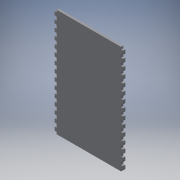
# Autodesk Inventor part: дно
Saved by Autodesk Inventor 2019 (Build 230136000, 136)
## iProperties
Created: 2022-02-24
Part Number: дно
Material: Типовые
Document SubType Name: Modeling
Designer: korsh
Density: 1 g/cm^3
Appearance: По умолчанию
Author: korsh
Autodesk Inventor part; units mm, degrees
ref_plane "YZ Plane" through (0, 0, 0) normal (1, 0, 0) x (0, 1, 0)
ref_plane "XZ Plane" through (0, 0, 0) normal (0, 1, 0) x (-1, 0, 0)
ref_plane "XY Plane" through (0, 0, 0) normal (0, 0, 1) x (1, 0, 0)
sketch "Эскиз1" plane through (0, 0, 0) normal (0, 0, 1) x (1, 0, 0)
  line L0 (0, 180) -> (0, 170) projected
  line L1 (0, 180) -> (-6, 180) projected
  line L2 (-6, 170) -> (-6, 180) projected
  line L3 (0, 170) -> (-6, 170) projected
  line L4 (0, 160) -> (0, 150) projected
  line L5 (0, 160) -> (-6, 160) projected
  line L6 (-6, 150) -> (-6, 160) projected
  line L7 (0, 150) -> (-6, 150) projected
  line L8 (0, 140) -> (0, 130) projected
  line L9 (0, 140) -> (-6, 140) projected
  line L10 (-6, 130) -> (-6, 140) projected
  line L11 (0, 130) -> (-6, 130) projected
  line L12 (0, 120) -> (0, 110) projected
  line L13 (0, 120) -> (-6, 120) projected
  line L14 (-6, 110) -> (-6, 120) projected
  line L15 (0, 110) -> (-6, 110) projected
  line L16 (0, 100) -> (0, 90) projected
  line L17 (0, 100) -> (-6, 100) projected
  line L18 (-6, 90) -> (-6, 100) projected
  line L19 (0, 90) -> (-6, 90) projected
  line L20 (0, 80) -> (0, 70) projected
  line L21 (0, 80) -> (-6, 80) projected
  line L22 (-6, 70) -> (-6, 80) projected
  line L23 (0, 70) -> (-6, 70) projected
  line L24 (0, 60) -> (0, 50) projected
  line L25 (0, 60) -> (-6, 60) projected
  line L26 (-6, 50) -> (-6, 60) projected
  line L27 (0, 50) -> (-6, 50) projected
  line L28 (0, 40) -> (0, 30) projected
  line L29 (0, 40) -> (-6, 40) projected
  line L30 (-6, 30) -> (-6, 40) projected
  line L31 (0, 30) -> (-6, 30) projected
  line L32 (0, 20) -> (0, 10) projected
  line L33 (0, 20) -> (-6, 20) projected
  line L34 (-6, 10) -> (-6, 20) projected
  line L35 (0, 10) -> (-6, 10) projected
  line L36 (0, 0) -> (0, -10) projected
  line L37 (0, 0) -> (-6, 0) projected
  line L38 (-6, -10) -> (-6, 0) projected
  line L39 (0, -10) -> (-6, -10) projected
  line L40 (0, -20) -> (0, -30) projected
  line L41 (0, -20) -> (-6, -20) projected
  line L42 (-6, -30) -> (-6, -20) projected
  line L43 (0, -30) -> (-6, -30) projected
  line L44 (0, -20) -> (0, -30) projected
  line L45 (0, -20) -> (-6, -20) projected
  line L46 (-6, -30) -> (-6, -20) projected
  line L47 (0, -30) -> (-6, -30) projected
  line L48 (0, -40) -> (0, -50) projected
  line L49 (0, -40) -> (-6, -40) projected
  line L50 (-6, -50) -> (-6, -40) projected
  line L51 (0, -50) -> (-6, -50) projected
  line L52 (0, -60) -> (0, -70) projected
  line L53 (0, -60) -> (-6, -60) projected
  line L54 (-6, -70) -> (-6, -60) projected
  line L55 (0, -70) -> (-6, -70) projected
  line L56 (0, -80) -> (0, -90) projected
  line L57 (0, -80) -> (-6, -80) projected
  line L58 (-6, -90) -> (-6, -80) projected
  line L59 (0, -90) -> (-6, -90) projected
  line L60 (0, -100) -> (0, -110) projected
  line L61 (0, -100) -> (-6, -100) projected
  line L62 (-6, -110) -> (-6, -100) projected
  line L63 (0, -110) -> (-6, -110) projected
  line L64 (-186, 180) -> (-186, 170) projected
  line L65 (-186, 180) -> (-192, 180) projected
  line L66 (-192, 170) -> (-192, 180) projected
  line L67 (-186, 170) -> (-192, 170) projected
  line L68 (-186, 160) -> (-186, 150) projected
  line L69 (-186, 160) -> (-192, 160) projected
  line L70 (-192, 150) -> (-192, 160) projected
  line L71 (-186, 150) -> (-192, 150) projected
  line L72 (-186, 140) -> (-186, 130) projected
  line L73 (-186, 140) -> (-192, 140) projected
  line L74 (-192, 130) -> (-192, 140) projected
  line L75 (-186, 130) -> (-192, 130) projected
  line L76 (-186, 120) -> (-186, 110) projected
  line L77 (-186, 120) -> (-192, 120) projected
  line L78 (-192, 110) -> (-192, 120) projected
  line L79 (-186, 110) -> (-192, 110) projected
  line L80 (-186, 100) -> (-186, 90) projected
  line L81 (-186, 100) -> (-192, 100) projected
  line L82 (-192, 90) -> (-192, 100) projected
  line L83 (-186, 90) -> (-192, 90) projected
  line L84 (-186, 80) -> (-186, 70) projected
  line L85 (-186, 80) -> (-192, 80) projected
  line L86 (-192, 70) -> (-192, 80) projected
  line L87 (-186, 70) -> (-192, 70) projected
  line L88 (-186, 60) -> (-186, 50) projected
  line L89 (-186, 60) -> (-192, 60) projected
  line L90 (-192, 50) -> (-192, 60) projected
  line L91 (-186, 50) -> (-192, 50) projected
  line L92 (-186, 20) -> (-186, 10) projected
  line L93 (-186, 20) -> (-192, 20) projected
  line L94 (-192, 10) -> (-192, 20) projected
  line L95 (-186, 10) -> (-192, 10) projected
  line L96 (-186, 40) -> (-186, 30) projected
  line L97 (-186, 40) -> (-192, 40) projected
  line L98 (-192, 30) -> (-192, 40) projected
  line L99 (-186, 30) -> (-192, 30) projected
  line L100 (-186, -20) -> (-186, -30) projected
  line L101 (-186, -20) -> (-192, -20) projected
  line L102 (-192, -30) -> (-192, -20) projected
  line L103 (-186, -30) -> (-192, -30) projected
  line L104 (-186, 0) -> (-186, -10) projected
  line L105 (-186, 0) -> (-192, 0) projected
  line L106 (-192, -10) -> (-192, 0) projected
  line L107 (-186, -10) -> (-192, -10) projected
  line L108 (-186, -40) -> (-186, -50) projected
  line L109 (-186, -40) -> (-192, -40) projected
  line L110 (-192, -50) -> (-192, -40) projected
  line L111 (-186, -50) -> (-192, -50) projected
  line L112 (-186, -60) -> (-186, -70) projected
  line L113 (-186, -60) -> (-192, -60) projected
  line L114 (-192, -70) -> (-192, -60) projected
  line L115 (-186, -70) -> (-192, -70) projected
  line L116 (-186, -80) -> (-186, -90) projected
  line L117 (-186, -80) -> (-192, -80) projected
  line L118 (-192, -90) -> (-192, -80) projected
  line L119 (-186, -90) -> (-192, -90) projected
  line L120 (-186, -100) -> (-186, -110) projected
  line L121 (-186, -100) -> (-192, -100) projected
  line L122 (-192, -110) -> (-192, -100) projected
  line L123 (-186, -110) -> (-192, -110) projected
  line L124 (-186, 186) -> (-186, 180) projected
  line L125 (-186, -110) -> (-186, -115.6956) projected
  line L126 (-6, 180) -> (-6, 186) projected
  line L127 (-6, -115.6956) -> (-6, -110) projected
  line L128 (-6, 186) -> (-186, 186)
  line L129 (-186, 186) -> (-186, -115.6956)
  line L130 (-186, -115.6956) -> (-6, -115.6956)
  line L131 (-6, -115.6956) -> (-6, 186)
  constraints: 8 end point, 2 parallel, 1 horizontal, 1 perpendicular
extrude "Выдавливание1" add sketch "Эскиз1" against normal blind 6
